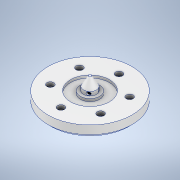
# Autodesk Inventor part: ODSY-0003-203
Saved by Autodesk Inventor 2021 (Build 250183000, 183)
## iProperties
Company: ERPL
Created: 2021-10-02
Material: Aluminum 6061
Document SubType Name: Modeling
Designer: WYATT ROBINSON
Density: 2.7 g/cm^3
Appearance: Aluminum - Flat
Mass: 136.745 g
Surface Area: 163.227 cm^2
Volume: 50.6463 cm^3
Project: ODYSSEY
Description: INJECTOR ELEMENT
Part Number: ODSY-0003-203
Author: WYATT ROBINSON
Revision Number: 00
Autodesk Inventor part; units mm, degrees
ref_plane "YZ Plane" through (0, 0, 0) normal (1, 0, 0) x (0, 1, 0)
ref_plane "XZ Plane" through (0, 0, 0) normal (0, 1, 0) x (-1, 0, 0)
ref_plane "XY Plane" through (0, 0, 0) normal (0, 0, 1) x (1, 0, 0)
sketch "Sketch1" plane through (0, 0, 0) normal (0, 1, 0) x (-1, 0, 0)
  circle A0 centre (0, 0) radius 19.05
  dimension "d0" = 38.1
  constraints: 1 centre point, 1 coincident
  measures "d0" diameter of A0
extrude "Extrusion1" add sketch "Sketch1" along normal blind 8.89
sketch "Sketch14" plane through (0, 0, 0) normal (0, -1, 0) x (1, 0, 0)
  circle A0 centre (0, 0) radius 19.05
  circle A1 centre (0, 0) radius 41.275
  circle A2 centre (0, 0) radius 19.05 projected
  dimension "d89" = 82.55
  constraints: 2 centre point, 2 coincident, 1 concentric
  measures "d89" diameter of A1
extrude "Extrusion7" add sketch "Sketch14" against normal blind 11.43
sketch "Sketch2" plane through (0, 0, 0) normal (0, -1, 0) x (1, 0, 0)
  point P0 (0, 0)
  point P1 (0, 28.575)
  dimension "d27" = 28.575
  constraints: 1 vertical alignment
  measures "d27" distance of point (0, 28.575) point (0, 0)
hole "Hole1" at (0, 0, 28.575) direction (0, 1, 0) diameter 6.7564 end through all counterbore diameter 12.7 counterbore depth 7.9375 clearance for "Socket Head Cap Screw" size "1/4" standard "Ansi Unified Screw Threads"
pattern_circular "Circular Pattern1" count 6 over 360 about axis through (0, -10, 0) along (0, 1, 0) of "Hole1"
sketch "Sketch4" plane through (0, 8.89, 0) normal (0, 1, 0) x (1, 0, 0)
  circle A0 centre (0, 0) radius 6.35
  dimension "d15" = 12.7
  constraints: 1 centre point, 1 coincident
  measures "d15" diameter of A0
extrude "Extrusion2" add sketch "Sketch4" along normal blind 6.35
sketch "Sketch5" plane through (0, 0, 0) normal (0, -1, 0) x (1, 0, 0)
  circle A0 centre (0, 0) radius 5.08
  dimension "d18" = 10.16
  constraints: 1 centre point, 1 coincident
  measures "d18" diameter of A0
extrude "Extrusion3" cut sketch "Sketch5" against normal through all
sketch "Sketch6" plane through (0, 0, 0) normal (1, 0, 0) x (0, 1, 0)
  line L0 (15.24, -6.35) -> (15.24, 6.35) projected
  line L1 (24.13, 0) -> (15.24, 0)
  line L2 (15.24, 6.35) -> (24.13, 1.27)
  line L3 (24.13, 1.27) -> (24.13, 0)
  point P0 (0, 0)
  dimension "d22" = 8.89
  dimension "d28" = 1.27
  constraints: 6 end point, 1 coincident, 1 horizontal, 1 midpoint, 1 vertical
  measures "d22" horizontal distance of L2.start L1.start
  measures "d28" distance of L2.end L1.start
revolve "Revolution1" add sketch "Sketch6" angle 360 about axis through (0, 24.13, 0) along (0, -1, 0)
sketch "Sketch7" plane through (0, 8.89, 0) normal (0, 1, 0) x (1, 0, 0)
  circle A0 centre (0, 0) radius 9.525
  circle A1 centre (0, 0) radius 6.35
  circle A2 centre (0, 0) radius 6.35 projected
  dimension "d24" = 19.05
  constraints: 2 centre point, 2 coincident, 1 concentric
  measures "d24" diameter of A0
extrude "Extrusion4" add sketch "Sketch7" along normal blind 2.54
sketch "Sketch8" plane through (0, 0, 0) normal (0, 0, 1) x (1, 0, 0)
  circle A0 centre (3.556, 13.335) radius 1.524
  line L0 (-5.08, 15.24) -> (5.08, 15.24) projected
  point P0 (0, 0)
  dimension "d29" = 3.048
  dimension "d30" = 1.905
  dimension "d31" = 3.556
  constraints: 1 centre point
  measures "d29" diameter of A0
  measures "d30" distance from line of L0 A0.centre
  measures "d31" horizontal distance of point (0, 0) A0.centre
extrude "Extrusion5" cut sketch "Sketch8" along normal through all
pattern_circular "Circular Pattern2" count 4 over 360 about axis through (0, 8.89, 0) along (0, 1, 0) of "Extrusion5"
chamfer "Chamfer4" distance 3.175 angle 45 1 edges at (-41.275, 0, 0)
body "Solid1"
